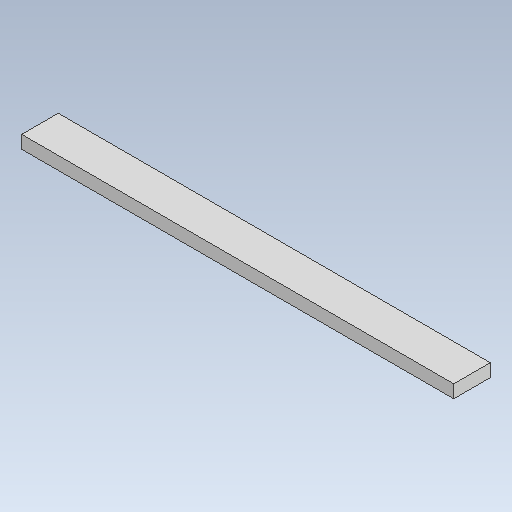
# Autodesk Inventor part: CENTREBUMP
Saved by Autodesk Inventor 2020 (Build 240168000, 168)
## iProperties
Created: 2021-01-07
Part Number: CENTREBUMP
Material: Generic
Document SubType Name: Modeling
Designer: lucky
Density: 1 g/cm^3
Appearance: Default
Mass: 1850.8 g
Surface Area: 1898.5 cm^2
Volume: 1850.8 cm^3
Author: lucky
Autodesk Inventor part; units mm, degrees
ref_plane "YZ Plane" through (0, 0, 0) normal (1, 0, 0) x (0, 1, 0)
ref_plane "XZ Plane" through (0, 0, 0) normal (0, 1, 0) x (-1, 0, 0)
ref_plane "XY Plane" through (0, 0, 0) normal (0, 0, 1) x (1, 0, 0)
sketch "Sketch1" plane through (0, 0, 0) normal (1, 0, 0) x (0, 1, 0)
  line L0 (-13.4938, -38.1) -> (13.4937, -38.1)
  line L1 (13.4937, -38.1) -> (13.4938, 38.1)
  line L2 (13.4938, 38.1) -> (-13.4937, 38.1)
  line L3 (-13.4937, 38.1) -> (-13.4938, -38.1)
  line L4 (-13.4938, -38.1) -> (13.4938, 38.1) construction
  line L5 (13.4937, -38.1) -> (-13.4937, 38.1) construction
  point P0 (0, 0)
  dimension "d0" = 26.9875
  dimension "d1" = 76.2
  constraints: 12 end point, 2 midpoint, 2 parallel, 1 horizontal, 1 perpendicular
  measures "d0" distance between parallel lines of L3 L1
  measures "d1" distance between parallel lines of L0 L2
extrude "Extrusion1" add sketch "Sketch1" against normal blind 900
body "Solid1"
